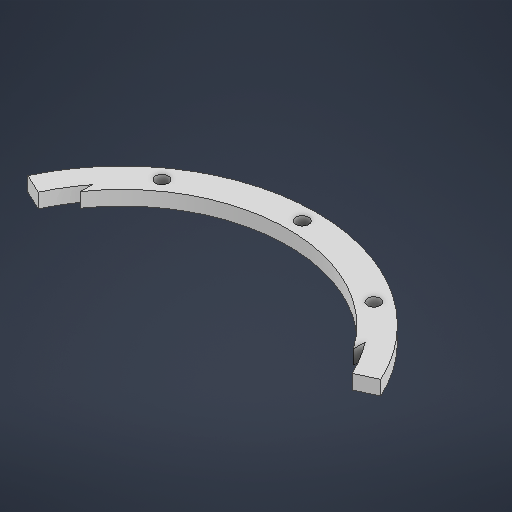
# Autodesk Inventor part: Camera Mount
Saved by Autodesk Inventor 2025 (Build 290162000, 162)
## iProperties
Created: 2024-10-25
Part Number: Camera Mount
Material: Generic
Document SubType Name: Modeling
Designer: mayhe
Density: 1 g/cm^3
Appearance: Default
Author: mayhe
Autodesk Inventor part; units mm, degrees
ref_plane "YZ Plane" through (0, 0, 0) normal (1, 0, 0) x (0, 1, 0)
ref_plane "XZ Plane" through (0, 0, 0) normal (0, 1, 0) x (-1, 0, 0)
ref_plane "XY Plane" through (0, 0, 0) normal (0, 0, 1) x (1, 0, 0)
sketch "Sketch1" plane through (0, 0, 0) normal (0, 1, 0) x (-1, 0, 0)
  circle A0 centre (0, 0) radius 135
  circle A1 centre (0, 0) radius 120
  circle A2 centre (0, 0) radius 125
  circle A3 centre (0, -125) radius 2.75
  circle A4 centre (0, -125) radius 4.45
  circle A5 centre (73.4732, -101.1271) radius 2.75
  circle A6 centre (73.4732, -101.1271) radius 4.45
  circle A7 centre (118.8821, -38.6271) radius 2.75
  circle A8 centre (118.8821, -38.6271) radius 4.45
  circle A9 centre (118.8821, 38.6271) radius 2.75
  circle A10 centre (118.8821, 38.6271) radius 4.45
  circle A11 centre (73.4732, 101.1271) radius 2.75
  circle A12 centre (73.4732, 101.1271) radius 4.45
  circle A13 centre (0, 125) radius 2.75
  circle A14 centre (0, 125) radius 4.45
  circle A15 centre (-73.4732, 101.1271) radius 2.75
  circle A16 centre (-73.4732, 101.1271) radius 4.45
  circle A17 centre (-118.8821, 38.6271) radius 2.75
  circle A18 centre (-118.8821, 38.6271) radius 4.45
  circle A19 centre (-118.8821, -38.6271) radius 2.75
  circle A20 centre (-118.8821, -38.6271) radius 4.45
  circle A21 centre (-73.4732, -101.1271) radius 2.75
  circle A22 centre (-73.4732, -101.1271) radius 4.45
  line L0 (0, 0) -> (199.3877, -92.976)
  line L1 (0, 0) -> (220, 0) construction
  line L2 (0, 0) -> (-199.3877, -92.976)
  line L3 (0, 0) -> (220, 0) construction
  circle A23 centre (0, 0) radius 115.125
  line L4 (-94.5, -15) -> (94.5, -15)
  line L5 (94.5, -15) -> (94.5, -235)
  line L6 (94.5, -235) -> (-94.5, -235)
  line L7 (-94.5, -235) -> (-94.5, -15)
  line L8 (-94.5, -15) -> (94.5, -235) construction
  line L9 (94.5, -15) -> (-94.5, -235) construction
  point P0 (-122.3516, -57.0535)
  point P1 (122.3516, -57.0535)
  point P2 (108.7569, -50.7142)
  point P3 (94.5, -73.9578)
  point P4 (94.5, -65.7534)
  point P5 (-94.5, -65.7534)
  point P6 (-94.5, -73.9578)
  point P7 (-108.7569, -50.7142)
  dimension "d2" = 250
  dimension "d0" = 270
  dimension "d1" = 240
  dimension "d3" = 5.5
  dimension "d4" = 8.9
  dimension "d7" = 360
  dimension "d11" = 220
  dimension "d12" = 25
  dimension "d13" = 220
  dimension "d14" = 155
  dimension "d15" = 230.25
  dimension "d16" = 189
  dimension "d17" = 220
  constraints: 23 centre point, 20 end point, 16 coincident, 3 horizontal, 2 equal length, 2 midpoint, 2 parallel, 1 perpendicular, 1 vertical alignment, 43 other
  measures "d0" diameter of A0
  measures "d1" diameter of A1
  measures "d3" diameter of A3
  measures "d4" diameter of A4
  measures "d11" distance of L0.start L0.end
  measures "d12" angle of L0 L1
  measures "d13" distance of L0.start L2.end
  measures "d14" angle of L2 L3
  measures "d15" diameter of A23
  measures "d16" distance of L5.end L6.end
  measures "d17" distance of L4.end L5.end
extrude "Extrusion1" add sketch "Sketch1" along normal blind 10 contours L2 A2 L7 A0 | A0 L5 A2 L0 | L7 A2 A22 A4 A6 L5 A0 | L2 A1 L7 A2 | A2 L5 A1 L0 | L7 A1 L5 A2 A6 A4 A22 | L7 A23 L5 A1
body "Solid1"
